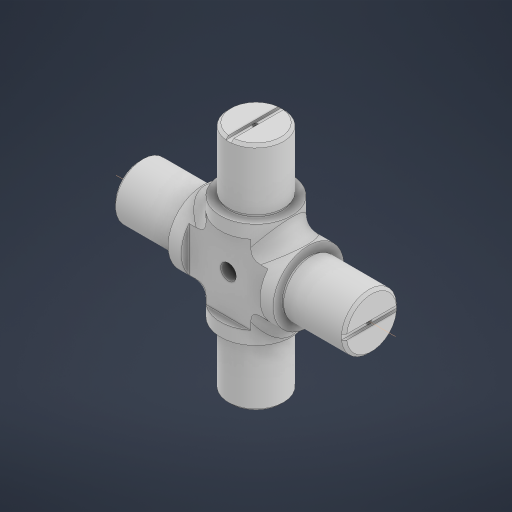
# Autodesk Inventor part: Part1
Saved by Autodesk Inventor 2023 (Build 270158000, 158)
## iProperties
Created: 2022-11-25
Part Number: Part1
Material: Generic
Document SubType Name: Modeling
Designer: iusti
Density: 1 g/cm^3
Appearance: Default
Author: iusti
Autodesk Inventor part; units mm, degrees
sketch "Sketch1" plane through (0, 0, 0) normal (1, 0, 0) x (0, 1, 0)
  circle A0 centre (0, 0) radius 13.5
  dimension "d0" = 27
  constraints: 1 centre point, 1 coincident
  measures "d0" diameter of A0
extrude "Extrusion1" add sketch "Sketch1" along normal mid plane 40
sketch "Sketch2" plane through (0, 0, 0) normal (0, 1, 0) x (-1, 0, 0)
  circle A0 centre (0, 0) radius 13.5
  dimension "d3" = 27
  constraints: 1 centre point, 1 coincident
  measures "d3" diameter of A0
extrude "Extrusion2" add sketch "Sketch2" along normal mid plane 40
fillet "Fillet1" radius 6 7 edges at (9.5459, 9.5459, 9.5459) (13.5, -13.5, 0) (9.5459, 9.5459, -9.5459) (-9.5459, 9.5459, 9.5459) (-9.5459, 9.5459, -9.5459) (-9.5459, -9.5459, 9.5459) (-9.5459, -9.5459, -9.5459)
sketch "Sketch3" plane through (0, 0, 0) normal (0, 0, 1) x (1, 0, 0)
  line L0 (-20, 13.5) -> (-20, -13.5) projected
  line L1 (-20, 10) -> (-21, 10)
  line L2 (-21, 10) -> (-21, 10.5)
  line L3 (-21, 10.5) -> (-44, 10.5)
  line L4 (-44, 10.5) -> (-44, 0)
  line L5 (-44, 0) -> (-20, 0)
  point P0 (0, 0)
  dimension "d7" = 21
  dimension "d8" = 24
  dimension "d9" = 1
  dimension "d10" = 20
  constraints: 8 end point, 3 perpendicular, 1 horizontal, 1 horizontal alignment, 1 midpoint, 1 point on line, 2 other
  measures "d8" distance between parallel lines of L0 L4
  measures "d9" distance of L1.start L1.end
revolve "Revolution1" add sketch "Sketch3" angle 360 about axis through (-44, 0, 0) along (1, 0, 0)
sketch "Sketch4" plane through (0, 0, 0) normal (0, 0, 1) x (1, 0, 0)
  line L0 (-44, -10.5) -> (-44, 10.5) projected
  line L1 (-56.8, 0) -> (32.8, 0) projected
  line L2 (-44, 1) -> (-43, 1)
  line L3 (-43, 1) -> (-43, -1)
  line L4 (-43, -1) -> (-44, -1)
  line L5 (-44, -1) -> (-44, 1)
  point P0 (0, 0)
  point P1 (-44, 0)
  dimension "d15" = 1
  dimension "d16" = 2
  constraints: 8 end point, 2 parallel, 1 collinear, 1 horizontal, 1 midpoint, 1 perpendicular, 1 point on line
  measures "d15" distance of L3.end L4.end
  measures "d16" distance of L2.end L3.end
extrude "Extrusion3" cut sketch "Sketch4" along normal mid plane 40
chamfer "Chamfer1" distance 1 angle 45 3 edges at (-44, 7.7701, 7.0622) (-44, 7.7701, -7.0622) (-44, -10.5, 0)
ref_plane "Work Plane2" through (0, 0, 0) normal (-0.7071068, 0.7071068, 0) x (0, 0, 1)
mirror "Mirror1" about plane through (0, 0, 0) normal (-0.7071068, 0.7071068, 0) of "Revolution1", "Extrusion3", "Chamfer1"
ref_plane "Work Plane3" through (0, 0, 0) normal (0.7071068, 0.7071068, 0) x (0, 0, 1)
mirror "Mirror2" about plane through (0, 0, 0) normal (0.7071068, 0.7071068, 0) of "Revolution1", "Extrusion3", "Chamfer1", "Mirror1"
ref_plane "Work Plane4" through (0, 0, 10.5) normal (0, 0, 1) x (1, 0, 0)
sketch "Sketch5" plane through (0, 0, 10.5) normal (0, 0, 1) x (1, 0, 0)
  line L0 (-15, -15) -> (15, -15)
  line L1 (15, -15) -> (15, 15)
  line L2 (15, 15) -> (-15, 15)
  line L3 (-15, 15) -> (-15, -15)
  line L4 (-19.5, -13.5) -> (0, 0) projected
  line L5 (-15, -15) -> (15, 15) construction
  line L6 (15, -15) -> (-15, 15) construction
  dimension "d25" = 30
  dimension "d26" = 30
  constraints: 12 end point, 2 midpoint, 2 parallel, 1 horizontal, 1 perpendicular
  measures "d25" distance of L2.end L1.end
  measures "d26" distance of L1.end L0.end
extrude "Extrusion4" cut sketch "Sketch5" along normal blind 40
mirror "Mirror3" about plane through (0, 0, 0) normal (0, 0, 1) of "Extrusion4"
sketch "Sketch6" plane through (0, 0, 10.5) normal (0, 0, 1) x (1, 0, 0)
  point P0 (0, 0)
hole "Hole1" at (0, 0, 10.5) direction (0, 0, -1) diameter 6 end through all
sketch "Sketch7" plane through (0, 43, 0) normal (0, 1, 0) x (1, 0, 0)
  arc A0 (-1, -10.4523) -> (1, -10.4523) centre (0, 0) ccw projected
hole "Hole2" at (0, 43, 0) direction (0, -1, 0) diameter 2 end through all
sketch "Sketch8" plane through (43, 0, 0) normal (1, 0, 0) x (0, 0, -1)
  arc A0 (10.4523, -1) -> (10.4523, 1) centre (0, 0) ccw projected
hole "Hole3" at (43, 0, 0) direction (-1, 0, 0) diameter 2 end through all
body "Solid1"
